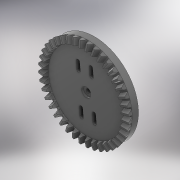
# Autodesk Inventor part: Bevel Gear2
Saved by Autodesk Inventor 2020.3 (Build 243373000, 373)
## iProperties
CustomPartVersion: 1
Created: 2021-08-24
Part Number: Bevel Gear2
Material: ABS Plastic
Document SubType Name: Modeling
Designer: justi
Categories: <?xml version="1.0" encoding="UTF-16"?> <MemberInstance><Categories><FamilyTemplate><FamilyTemplateParameter ValueType="xs:double" Id="1" ObjectReferenceKey="da_z" ObjectType="kUserParameterObject"/><FamilyTemplateParameter ValueType="xs:double" Id="2" ObjectReferenceKey="da_b" ObjectType="kUserParameterObject"/><FamilyTemplateParameter ValueType="xs:double" Id="3" ObjectReferenceKey="da_beta" ObjectType="kUserParameterObject"/><FamilyTemplateParameter ValueType="xs:double" Id="4" ObjectReferenceKey="da_dae" ObjectType="kUserParameterObject"/><FamilyTemplateParameter ValueType="xs:double" Id="5" ObjectReferenceKey="da_ve" ObjectType="kUserParameterObject"/><FamilyTemplateParameter ValueType="xs:double" Id="6" ObjectReferenceKey="da_omega" ObjectType="kUserParameterObject"/><FamilyTemplateParameter ValueType="xs:string" Id="7" ObjectReferenceKey="EAIAABAAAAAAHwAAAAAAAIAAAAAAAAAA" ObjectType="83914240" SubObjectId="SurfaceGeometry"/></FamilyTemplate><ParamToTemplateMap><ParamToTemplate CategoryParameter="//CategoryParameter[@InternalName='046C89C9-8512-4d59-83FE-43B91F4F132A']" TemplateParameter="1"/><ParamToTemplate CategoryParameter="//CategoryParameter[@InternalName='2552DF32-E462-4b46-AEBF-C6C7768E72AC']" TemplateParameter="2"/><ParamToTemplate CategoryParameter="//CategoryParameter[@InternalName='C9EE641D-15FC-4fae-A226-E94C4372FDD7']" TemplateParameter="3"/><ParamToTemplate><ParamToTemplate CategoryParameter="//CategoryParameter[@InternalName='00B6519A-459B-49c7-AD84-2E56D39A5744']" ConstantValue="-0.000000"/></ParamToTemplate><ParamToTemplate><ParamToTemplate CategoryParameter="//CategoryParameter[@InternalName='04B31F0E-C7A6-4894-AA32-9629BEFACF47']" ConstantValue="1.000000"/></ParamToTemplate><ParamToTemplate><ParamToTemplate CategoryParameter="//CategoryParameter[@InternalName='43CBEC2E-7847-49e7-A936-2F7889FCB2D9']" ConstantValue="0.200000"/></ParamToTemplate><ParamToTemplate><ParamToTemplate CategoryParameter="//CategoryParameter[@InternalName='B1EFC894-105D-4ebd-86BF-FA20ED196853']" ConstantValue="0.300000"/></ParamToTemplate><ParamToTemplate><ParamToTemplate CategoryParameter="//CategoryParameter[@InternalName='51175063-3D10-4879-93E8-6246FE8B403D']" ConstantValue="2060000000.000000"/></ParamToTemplate><ParamToTemplate><ParamToTemplate CategoryParameter="//CategoryParameter[@InternalName='A3A52E27-4454-46a9-B0BD-C932399B70AF']" ConstantValue="0.300000"/></ParamToTemplate><ParamToTemplate CategoryParameter="//CategoryParameter[@InternalName='2A200944-5A8C-41ca-B96E-8520D2E510F1']" TemplateParameter="4"/><ParamToTemplate><ParamToTemplate CategoryParameter="//CategoryParameter[@InternalName='1A637F62-92C8-44bc-B81F-10802510B579']" ConstantValue="12.205961"/></ParamToTemplate><ParamToTemplate CategoryParameter="//CategoryParameter[@InternalName='B52DD4BE-6863-48fb-BF58-89EF6F9EC65C']" TemplateParameter="5"/><ParamToTemplate><ParamToTemplate CategoryParameter="//CategoryParameter[@InternalName='3956BFF2-84D2-457d-93C2-9B0613DEBA67']" ConstantValue="1.214973"/></ParamToTemplate><ParamToTemplate CategoryParameter="//CategoryParameter[@InternalName='739CFA02-461B-4bf8-8049-181FCAD8B28F']" TemplateParameter="6"/><ParamToTemplate><ParamToTemplate CategoryParameter="//CategoryParameter[@InternalName='A27E999F-E2CE-4481-8A2A-EBF499C4C3C5']" ConstantValue="-0.000000"/></ParamToTemplate><ParamToTemplate><ParamToTemplate CategoryParameter="//CategoryParameter[@InternalName='9E1B4470-B2D3-4ff1-B813-535BB4CDF51A']" ConstantValue="3520000.000000"/></ParamToTemplate><ParamToTemplate><ParamToTemplate CategoryParameter="//CategoryParameter[@InternalName='F8452263-BFF6-458c-9FB1-07C4B99E95CD']" ConstantValue="11400000.000000"/></ParamToTemplate><ParamToTemplate><ParamToTemplate CategoryParameter="//CategoryParameter[@InternalName='3E3BB259-FD49-497f-8171-6EBC954A3479']" ConstantValue="2.000000"/></ParamToTemplate><ParamToTemplate CategoryParameter="//CategoryParameter[@InternalName='27C3BAF2-7550-4e4b-AE2C-0DB134B7D9B7']" TemplateParameter="7"/></ParamToTemplateMap><Category DisplayName="Gear" InternalName="DC85795E-93AB-48d5-8EEE-5A27447B64BD" Mnemonic="Gear"><CategoryParameter DisplayName="z" InternalName="046C89C9-8512-4d59-83FE-43B91F4F132A" Mnemonic="z"/><CategoryParameter DisplayName="b" InternalName="2552DF32-E462-4b46-AEBF-C6C7768E72AC" Mnemonic="b"/><CategoryParameter DisplayName="||b|" InternalName="C9EE641D-15FC-4fae-A226-E94C4372FDD7" Mnemonic="beta"/><CategoryParameter DisplayName="x" InternalName="00B6519A-459B-49c7-AD84-2E56D39A5744" Mnemonic="x"/><CategoryParameter DisplayName="a*" InternalName="04B31F0E-C7A6-4894-AA32-9629BEFACF47" Mnemonic="a"/><CategoryParameter DisplayName="c*" InternalName="43CBEC2E-7847-49e7-A936-2F7889FCB2D9" Mnemonic="c"/><CategoryParameter DisplayName="r|.f|*" InternalName="B1EFC894-105D-4ebd-86BF-FA20ED196853" Mnemonic="rf"/><CategoryParameter DisplayName="E" InternalName="51175063-3D10-4879-93E8-6246FE8B403D" Mnemonic="E"/><CategoryParameter DisplayName="||m|" InternalName="A3A52E27-4454-46a9-B0BD-C932399B70AF" Mnemonic="mi"/><Category DisplayName="BevelGear" InternalName="0C98F69A-0C2B-4791-B2FE-7691BB227E77" Mnemonic="BevelGear"><CategoryParameter DisplayName="d|.ae|" InternalName="2A200944-5A8C-41ca-B96E-8520D2E510F1" Mnemonic="dae"/><CategoryParameter DisplayName="d|.ai|" InternalName="1A637F62-92C8-44bc-B81F-10802510B579" Mnemonic="dai"/><CategoryParameter DisplayName="A|.e|" InternalName="B52DD4BE-6863-48fb-BF58-89EF6F9EC65C" Mnemonic="ve"/><CategoryParameter DisplayName="A|.i|" InternalName="3956BFF2-84D2-457d-93C2-9B0613DEBA67" Mnemonic="vi"/><CategoryParameter DisplayName="||S|" InternalName="739CFA02-461B-4bf8-8049-181FCAD8B28F" Mnemonic="omega"/><CategoryParameter DisplayName="x|.t|" InternalName="A27E999F-E2CE-4481-8A2A-EBF499C4C3C5" Mnemonic="xt"/><CategoryParameter DisplayName="||s||.Flim|" InternalName="9E1B4470-B2D3-4ff1-B813-535BB4CDF51A" Mnemonic="sFlim"/><CategoryParameter DisplayName="||s||.Hlim|" InternalName="F8452263-BFF6-458c-9FB1-07C4B99E95CD" Mnemonic="sHlim"/><CategoryParameter DisplayName="type" InternalName="3E3BB259-FD49-497f-8171-6EBC954A3479" Mnemonic="type"/><CategoryParameter DisplayName="PitchDiameter" InternalName="27C3BAF2-7550-4e4b-AE2C-0DB134B7D9B7" Mnemonic="IDS_PITCHDIAM"/></Category></Category></Categories></MemberInstance>
Mass: 60.9118 g
Surface Area: 34.3074 cm^2
Volume: 7.7496 cm^3
Density: 1.06 g/cm^3
Appearance: Smooth - Black
Author: justi
Autodesk Inventor part; units mm, degrees
ref_plane "Mesh Plane2" through (0, 0, 0) normal (0.9969173, 0.0784591, 0) x (0, 0, 1)
sketch "Teeth Body Sketch" plane through (0, 0, 0) normal (1, 0, 0) x (0, 1, 0)
  line L0 (0, 0) -> (68.98135, -21.574599) construction
  line L1 (68.98135, -21.574599) -> (70.848875, -14.104501)
  line L2 (70.848875, -14.104501) -> (0, 0) construction
  line L3 (70, -17.5) -> (0, 0) construction
  line L4 (59.421102, -18.584536) -> (61.029803, -12.149733)
  line L5 (68.98135, -21.574599) -> (59.421102, -18.584536)
  line L6 (70.848875, -14.104501) -> (61.029803, -12.149733)
  line L7 (0, -24.040267) -> (0, 4.006711)
  line L8 (0, -17.5) -> (70.848875, -17.5) construction
  dimension "d0" = 140
  dimension "d1" = 137.9627
  dimension "d2" = 141.69775
  dimension "d3" = 10
  dimension "d4" = 14.1045
  constraints: 16 end point, 4 point on line, 3 perpendicular, 2 collinear, 1 horizontal alignment, 1 vertical alignment
  measures "d0" diameter of L3.start L7
  measures "d1" diameter of L0.end L7
  measures "d2" diameter of L1.end L7
  measures "d3" distance between parallel lines of L1 L4
  measures "d4" vertical distance of L1.end L0.start
revolve "Teeth Body" add sketch "Teeth Body Sketch" angle 360 about axis through (0, 0, 0) along (0, 0, 1)
ref_plane "Tooth Plane" through (0, 70, -17.5) normal (0, -0.9701425, 0.2425356) x (1, 0, 0)
sketch "Start Sketch" plane through (0, 70, -17.5) normal (0, -0.9701425, 0.2425356) x (1, 0, 0)
  line L0 (0, -322.683842) -> (0, 60.090014)
  arc A0 (-1.095494, -5.124) -> (-5.063259, 5.766461) centre (-96.817893, -33.830903) ccw
  arc A1 (5.063259, 5.766461) -> (1.095494, -5.124) centre (96.817893, -33.830903) ccw
  line L1 (-1.095494, -5.124) -> (1.095494, -5.124)
  arc A2 (5.063259, 5.766461) -> (-5.063259, 5.766461) centre (0, -288.617394) ccw
  dimension "d7" = 99.9343
  dimension "d8" = 96.81789
  dimension "d9" = 254.78649
  dimension "d57" = 294.42739
  dimension "d58" = 283.49339
  constraints: 6 point on circle, 3 centre point, 3 symmetric about line, 2 end point, 1 coincident, 1 perpendicular, 1 other
  measures "d7" radius of A0
  measures "d8" horizontal distance of point (0, -288.617) A0.centre
  measures "d9" vertical distance of point (0, -288.617) A0.centre
  measures "d57" radius of A2
  measures "d58" distance from line of A2.centre L1
sketch "End Sketch" plane through (0, 59.92507, -14.981268) normal (0, -0.9701425, 0.2425356) x (1, 0, 0)
  line L0 (0, -272.800641) -> (0, 50.800787)
  arc A0 (-0.937822, -4.386515) -> (-4.334517, 4.936508) centre (-82.883129, -28.961704) ccw
  arc A1 (4.334517, 4.936508) -> (0.937822, -4.386515) centre (82.883129, -28.961704) ccw
  line L1 (-0.937822, -4.386515) -> (0.937822, -4.386515)
  arc A2 (4.334517, 4.936508) -> (-4.334517, 4.936508) centre (0, -247.077394) ccw
  dimension "d12" = 85.551
  dimension "d15" = 82.88313
  dimension "d16" = 218.11569
  dimension "d59" = 252.05117
  dimension "d60" = 242.69088
  constraints: 6 point on circle, 3 centre point, 3 symmetric about line, 2 end point, 1 coincident, 1 other
  measures "d12" radius of A0
  measures "d15" horizontal distance of A0.centre point (0, -247.077)
  measures "d16" vertical distance of A0.centre point (0, -247.077)
  measures "d59" radius of A2
  measures "d60" distance from line of A2.centre L1
loft "Loft" cut profiles "Start Sketch", "End Sketch"
pattern_circular "Circular Pattern" count 40 over 360 about axis through (0, 0, 0) along (0, 0, 1) of "Loft"
ref_plane "End Plane" through (0, 59.92507, -14.981268) normal (0, -0.9701425, 0.2425356) x (1, 0, 0)
sketch3d "3D Sketch Right"
ref_plane "End Plane Right" through (-1.818828, 59.897461, -14.981268) normal (0.0294455, -0.9696955, 0.2425356) x (0.9995393, 0.0303517, 0)
sketch "End Sketch Right" plane through (-1.818828, 59.897461, -14.981268) normal (0.0294455, -0.9696955, 0.2425356) x (0.9995393, 0.0303517, 0)
  arc A0 (-0.937822, -4.386515) -> (-4.334517, 4.936508) centre (-82.883129, -28.961704) ccw
  line L0 (0, -298.973145) -> (0, 56.467763)
  arc A1 (4.334517, 4.936508) -> (0.937822, -4.386515) centre (82.883129, -28.961704) ccw
  line L1 (-0.937822, -4.386515) -> (0.937822, -4.386515)
  arc A2 (4.334517, 4.936508) -> (-4.334517, 4.936508) centre (0, -247.077394) ccw
  dimension "d70" = 82.88313
  dimension "d71" = 218.11569
  dimension "d72" = 85.551
  dimension "d73" = 242.69088
  dimension "d74" = 252.05117
  constraints: 6 point on circle, 3 centre point, 3 symmetric about line, 2 end point, 1 coincident, 1 perpendicular, 1 other
  measures "d70" horizontal distance of A2.centre A0.centre
  measures "d71" vertical distance of point (0, -247.077) A0.centre
  measures "d72" radius of A0
  measures "d73" distance from line of point (0, -247.077) L1
  measures "d74" radius of A2
feature "Loft Right" [suppressed]
pattern_circular "Circular Pattern Right" [suppressed]
sketch3d "3D Sketch Left"
ref_plane "End Plane Left" through (1.837136, 59.897461, -14.99459) normal (-0.0297401, -0.9696363, 0.2427365) x (0.99953, -0.0306569, 0)
sketch "End Sketch Left" plane through (1.837136, 59.897461, -14.99459) normal (-0.0297401, -0.9696363, 0.2427365) x (0.99953, -0.0306569, 0)
  line L0 (0, -298.977174) -> (0, 56.496282)
  arc A0 (-0.937822, -4.373722) -> (-4.334517, 4.949301) centre (-82.883129, -28.94891) ccw
  arc A1 (4.334517, 4.949301) -> (0.937822, -4.373722) centre (82.883129, -28.94891) ccw
  line L1 (-0.937822, -4.373722) -> (0.937822, -4.373722)
  ellipse E0 centre (0, -11.786362) end of major axis (61.029803, -11.786362) minor radius 14.814159
  arc A2 (4.334517, 4.949301) -> (-4.334517, 4.949301) centre (0, -247.0646) ccw
  dimension "d56" = 14.81416
  dimension "d30" = 85.551
  dimension "d31" = 82.88313
  dimension "d32" = 218.11569
  dimension "d61" = 252.05117
  dimension "d62" = 242.69088
  constraints: 6 point on circle, 3 centre point, 3 symmetric about line, 2 end point, 1 coincident, 2 other
  measures "d30" radius of A0
  measures "d31" horizontal distance of point (0, -247.065) A0.centre
  measures "d32" vertical distance of A0.centre point (0, -247.065)
  measures "d61" radius of A2
  measures "d62" distance from line of point (0, -247.065) L1
feature "Loft Left" [suppressed]
pattern_circular "Circular Pattern Left" [suppressed]
sketch "Body Sketch" plane through (0, 0, 0) normal (1, 0, 0) x (0, 1, 0)
  line L0 (0, -20.631568) -> (0, -16.445481)
  line L1 (68.98135, -21.574599) -> (59.421102, -18.584536)
  line L2 (59.421102, -18.584536) -> (0, -18.584536)
  line L3 (68.98135, -21.574599) -> (0, -21.574599)
  constraints: 4 end point, 2 perpendicular, 2 point on line
sketch "Body Sketch outline for Fix Body" plane through (0, 0, 0) normal (1, 0, 0) x (0, 1, 0)
  line L0 (0, -21.574599) -> (68.98135, -21.574599)
  line L1 (0, -18.584536) -> (0, -21.574599)
  line L2 (59.421102, -18.584536) -> (0, -18.584536)
  line L3 (68.98135, -21.574599) -> (59.421102, -18.584536)
revolve "Fix Body" add sketch "Body Sketch outline for Fix Body" angle 360 about axis through (0, 0, 0) along (0, 0, 1)
sketch "Sketch6" plane through (0, 0, 0) normal (1, 0, 0) x (0, 1, 0)
  line L0 (70, -17.5) -> (0, 0) projected
  line L1 (0, -19.5) -> (0, 3.25) projected
surface revolve "Pitch Diameter" sketch "Sketch6" angle 360 about axis through (0, 0, 0) along (0, 0, 1) shown no curves L0
sketch "Sketch8" plane through (0, 0, -40.829907) normal (0, 0, -1) x (-0.9973374, 0.0729256, 0)
  arc A0 (3.133653, 69.514451) -> (-6.611178, 69.270275) centre (0, 0) ccw
  circle A1 centre (0, 0) radius 69.585047
  point P0 (-6.700633, 126.311513)
  point P1 (-4.095775, 77.208157)
  constraints: 1 centre point, 1 coincident, 1 point on circle
extrude "Extrusion1" [suppressed]
sketch "Sketch9" plane through (0, 0, -21.574599) normal (0, 0, -1) x (-0.9969173, 0.0784591, 0)
  arc A0 (66.740837, 17.438101) -> (64.24433, 25.12156) centre (0, 0) ccw
  circle A1 centre (0, 0) radius 68.98135
  constraints: 1 coincident, 3 other
extrude "Extrusion2" add sketch "Sketch9" along normal blind 10
sketch "Sketch10" plane through (0, 0, -18.584536) normal (0, 0, 1) x (0.9969173, 0.0784591, 0)
  line L0 (13, -30.5) -> (13, 30.5) construction
  line L1 (13, 30.5) -> (-13, 30.5) construction
  line L2 (-13, 30.5) -> (-13, -30.5) construction
  line L3 (-13, -30.5) -> (13, -30.5) construction
  line L4 (13, -30.5) -> (-13, 30.5) construction
  line L5 (13, 30.5) -> (-13, -30.5) construction
  line L6 (-13, -30.5) -> (-10.25, -30.5)
  line L7 (-13, 30.5) -> (-10.25, 30.5)
  line L8 (13, -30.5) -> (10.25, -30.5) construction
  line L9 (13, 30.5) -> (10.25, 30.5)
  line L10 (10.25, -36.5) -> (10.25, -24.5) construction
  line L11 (13, -36.5) -> (13, -24.5)
  line L12 (7.5, -24.5) -> (7.5, -36.5)
  arc A0 (7.5, -36.5) -> (13, -36.5) centre (10.25, -36.5) ccw
  arc A1 (13, -24.5) -> (7.5, -24.5) centre (10.25, -24.5) ccw
  arc A2 (-13, -36.5) -> (-7.5, -36.5) centre (-10.25, -36.5) ccw
  line L13 (-13, -24.5) -> (-13, -36.5)
  line L14 (-7.5, -36.5) -> (-7.5, -24.5)
  arc A3 (-7.5, -24.5) -> (-13, -24.5) centre (-10.25, -24.5) ccw
  arc A4 (7.5, 24.5) -> (13, 24.5) centre (10.25, 24.5) ccw
  line L15 (7.5, 36.5) -> (7.5, 24.5)
  line L16 (13, 24.5) -> (13, 36.5)
  arc A5 (13, 36.5) -> (7.5, 36.5) centre (10.25, 36.5) ccw
  arc A6 (-13, 24.5) -> (-7.5, 24.5) centre (-10.25, 24.5) ccw
  line L17 (-13, 36.5) -> (-13, 24.5)
  line L18 (-7.5, 24.5) -> (-7.5, 36.5)
  arc A7 (-7.5, 36.5) -> (-13, 36.5) centre (-10.25, 36.5) ccw
  point P0 (0, 0)
  point P1 (0, 0)
  point P2 (0, 0)
  dimension "d98" = 61
  dimension "d99" = 26
  dimension "d100" = 2.75
  dimension "d101" = 2.75
  dimension "d102" = 2.75
  dimension "d103" = 2.75
  dimension "d104" = 6
  dimension "d105" = 5.5
  dimension "d106" = 6
  dimension "d107" = 5.5
  dimension "d108" = 6
  dimension "d109" = 5.5
  dimension "d110" = 6
  dimension "d111" = 5.5
  constraints: 40 end point, 16 point on circle, 16 tangent, 8 centre point, 6 parallel, 4 point on line, 3 midpoint, 2 vertical, 1 coincident, 1 perpendicular
  measures "d98" distance of L0.start L0.end
  measures "d99" distance of L1.end L0.end
  measures "d100" distance of L2.end L6.end
  measures "d101" distance of L1.end L7.end
  measures "d102" distance of L0.start L8.end
  measures "d103" distance of L0.end L9.end
  measures "d104" distance of L8.end L10.end
  measures "d105" diameter of A1
  measures "d106" distance of point (-10.25, -30.5) A3.centre
  measures "d107" diameter of A3
  measures "d108" distance of point (10.25, 30.5) A5.centre
  measures "d109" diameter of A5
  measures "d110" distance of point (-10.25, 30.5) A7.centre
  measures "d111" diameter of A7
extrude "Extrusion3" cut sketch "Sketch10" against normal through all
sketch "Sketch12" plane through (0, 0, -31.574599) normal (0, 0, -1) x (-1, 0, 0)
  circle A0 centre (0, 0) radius 7.275
  line L0 (7.275, 0) -> (-7.275, 0) construction
  line L1 (0, 7.275) -> (0, -7.275) construction
  line L2 (9.775, 2.5) -> (4.775, 2.5)
  line L3 (4.775, 2.5) -> (4.775, -2.5)
  line L4 (4.775, -2.5) -> (9.775, -2.5)
  line L5 (9.775, -2.5) -> (9.775, 2.5)
  line L6 (9.775, 2.5) -> (4.775, -2.5) construction
  line L7 (4.775, 2.5) -> (9.775, -2.5) construction
  line L8 (2.5, 9.775) -> (-2.5, 9.775)
  line L9 (-2.5, 9.775) -> (-2.5, 4.775)
  line L10 (-2.5, 4.775) -> (2.5, 4.775)
  line L11 (2.5, 4.775) -> (2.5, 9.775)
  line L12 (2.5, 9.775) -> (-2.5, 4.775) construction
  line L13 (-2.5, 9.775) -> (2.5, 4.775) construction
  line L14 (-9.775, 2.5) -> (-4.775, 2.5)
  line L15 (-4.775, 2.5) -> (-4.775, -2.5)
  line L16 (-4.775, -2.5) -> (-9.775, -2.5)
  line L17 (-9.775, -2.5) -> (-9.775, 2.5)
  line L18 (-9.775, 2.5) -> (-4.775, -2.5) construction
  line L19 (-4.775, 2.5) -> (-9.775, -2.5) construction
  line L20 (-2.5, -4.775) -> (2.5, -4.775)
  line L21 (2.5, -4.775) -> (2.5, -9.775)
  line L22 (2.5, -9.775) -> (-2.5, -9.775)
  line L23 (-2.5, -9.775) -> (-2.5, -4.775)
  line L24 (-2.5, -4.775) -> (2.5, -9.775) construction
  line L25 (2.5, -4.775) -> (-2.5, -9.775) construction
  point P0 (6.831956, 2.5)
  point P1 (2.5, 6.831956)
  point P2 (-2.5, 6.831956)
  point P3 (-6.831956, 2.5)
  point P4 (-6.831956, -2.5)
  point P5 (-2.5, -6.831956)
  point P6 (2.5, -6.831956)
  point P7 (6.831956, -2.5)
  dimension "d143" = 14.55
  dimension "d141" = 5
  dimension "d142" = 5
  dimension "d139" = 5
  dimension "d140" = 5
  dimension "d137" = 5
  dimension "d138" = 5
  dimension "d135" = 5
  dimension "d136" = 5
  constraints: 52 end point, 8 midpoint, 8 parallel, 5 horizontal, 5 perpendicular, 4 point on circle, 1 centre point, 1 coincident
  measures "d143" diameter of A0
  measures "d141" distance of L4.end L3.end
  measures "d142" distance of L3.end L2.end
  measures "d139" distance of L10.end L9.end
  measures "d140" distance of L9.end L8.end
  measures "d137" distance of L15.end L16.end
  measures "d138" distance of L14.end L15.end
  measures "d135" distance of L21.end L22.end
  measures "d136" distance of L20.end L21.end
extrude "Extrusion4" add sketch "Sketch12" along normal blind 5 contours L2 L3 L4 A0 L21 L20 L23 L16 L15 L14 L9 L10 L11
sketch "Sketch13" plane through (0, 0, -18.584536) normal (0, 0, 1) x (0.9969173, 0.0784591, 0)
  line L0 (13, -30.5) -> (13, 30.5) construction
  line L1 (13, 30.5) -> (-13, 30.5) construction
  line L2 (-13, 30.5) -> (-13, -30.5) construction
  line L3 (-13, -30.5) -> (13, -30.5) construction
  line L4 (13, -30.5) -> (-13, 30.5) construction
  line L5 (13, 30.5) -> (-13, -30.5) construction
  line L6 (-13, -30.5) -> (-10.25, -30.5)
  line L7 (-13, 30.5) -> (-10.25, 30.5)
  line L8 (13, -30.5) -> (10.25, -30.5) construction
  line L9 (13, 30.5) -> (10.25, 30.5)
  line L10 (10.25, -36.5) -> (10.25, -24.5) construction
  line L11 (13, -36.5) -> (13, -24.5)
  line L12 (7.5, -24.5) -> (7.5, -36.5)
  arc A0 (7.5, -36.5) -> (13, -36.5) centre (10.25, -36.5) ccw
  arc A1 (13, -24.5) -> (7.5, -24.5) centre (10.25, -24.5) ccw
  arc A2 (-13, -36.5) -> (-7.5, -36.5) centre (-10.25, -36.5) ccw
  line L13 (-13, -24.5) -> (-13, -36.5)
  line L14 (-7.5, -36.5) -> (-7.5, -24.5)
  arc A3 (-7.5, -24.5) -> (-13, -24.5) centre (-10.25, -24.5) ccw
  arc A4 (7.5, 24.5) -> (13, 24.5) centre (10.25, 24.5) ccw
  line L15 (7.5, 36.5) -> (7.5, 24.5)
  line L16 (13, 24.5) -> (13, 36.5)
  arc A5 (13, 36.5) -> (7.5, 36.5) centre (10.25, 36.5) ccw
  arc A6 (-13, 24.5) -> (-7.5, 24.5) centre (-10.25, 24.5) ccw
  line L17 (-13, 36.5) -> (-13, 24.5)
  line L18 (-7.5, 24.5) -> (-7.5, 36.5)
  arc A7 (-7.5, 36.5) -> (-13, 36.5) centre (-10.25, 36.5) ccw
  point P0 (0, 0)
  point P1 (0, 0)
  dimension "d161" = 61
  dimension "d160" = 26
  dimension "d159" = 2.75
  dimension "d158" = 2.75
  dimension "d157" = 2.75
  dimension "d156" = 2.75
  dimension "d155" = 6
  dimension "d154" = 5.5
  dimension "d152" = 6
  dimension "d153" = 5.5
  dimension "d150" = 6
  dimension "d151" = 5.5
  dimension "d148" = 6
  dimension "d149" = 5.5
  constraints: 40 end point, 16 point on circle, 16 tangent, 8 centre point, 6 parallel, 4 point on line, 3 midpoint, 2 vertical, 1 coincident, 1 perpendicular
  measures "d161" distance of L0.start L0.end
  measures "d160" distance of L1.end L0.end
  measures "d159" distance of L2.end L6.end
  measures "d158" distance of L1.end L7.end
  measures "d157" distance of L0.start L8.end
  measures "d156" distance of L0.end L9.end
  measures "d155" distance of L8.end L10.end
  measures "d154" diameter of A1
  measures "d152" distance of point (-10.25, -30.5) A3.centre
  measures "d153" diameter of A3
  measures "d150" distance of point (10.25, 30.5) A5.centre
  measures "d151" diameter of A5
  measures "d148" distance of point (-10.25, 30.5) A7.centre
  measures "d149" diameter of A7
hole "Hole2" at (0, 0, -18.584536) direction (0, 0, -1) diameter 6.6 end through all counterbore diameter 14.55 counterbore depth 3
equation "\"d0\" = da_de"
equation "\"d1\" = da_dfe"
equation "\"d2\" = da_dae"
equation "\"d3\" = da_b"
equation "\"d4\" = da_ve"
equation "\"d7\" = fd_rr"
equation "\"d8\" = fd_x"
equation "\"d9\" = fd_y"
equation "\"d57\" = 0.5 * fd_dva + 0.3 * da_he"
equation "\"d58\" = 0.5 * fd_dva - 1.12 * da_he"
equation "\"da_teethtype\" = 0"
equation "\"da_b\" = 10"
equation "\"da_de\" = 140"
equation "\"da_dae\" = 141.69775"
equation "\"da_dfe\" = 137.9627"
equation "\"da_le\" = 72.15435"
equation "\"da_omega\" = 90deg"
equation "\"da_beta\" = 0"
equation "\"da_delta\" = 75.963757deg"
equation "\"da_alpha\" = 20deg"
equation "\"da_he\" = 7.7"
equation "\"da_ve\" = 14.1045"
equation "\"da_zv\" = 164.924225"
equation "\"fd_loft\" = da_b + 0.05 * da_he"
equation "\"fd_x\" = fd_x1 + fd_x2"
equation "\"fd_y\" = fd_y1 - fd_y2"
equation "\"fd_dd\" = fd_dva - 0.8 * da_he"
equation "\"da_dvw\" = 577.23479"
equation "\"d11\" = fd_loft"
equation "\"da_dm\" = 130.29857"
equation "\"da_x\" = 0"
equation "\"da_m\" = 3.5"
equation "\"d50\" = da_omega"
equation "\"fd_rr\" = 99.934298"
equation "\"fd_dva\" = 584.234788"
equation "\"fd_x1\" = 2.779394"
equation "\"fd_x2\" = 94.038499"
equation "\"fd_y1\" = 288.604011"
equation "\"fd_y2\" = 33.81752"
body "Solid1"
body "Srf1"
